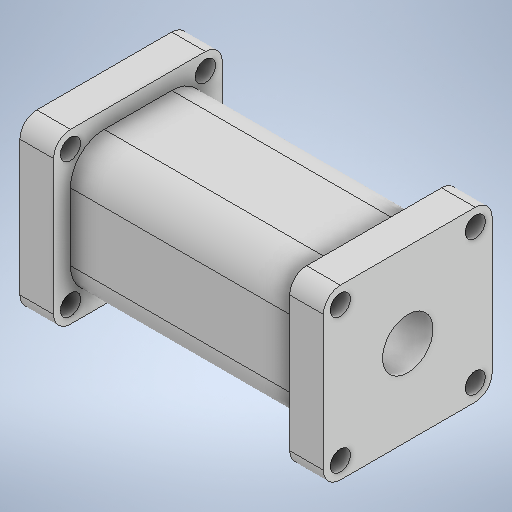
# Autodesk Inventor part: Contenedor
Saved by Autodesk Inventor 2025.1 (Build 291241000, 241)
## iProperties
Created: 2025-02-26
Part Number: Contenedor
Material: Generic
Document SubType Name: Modeling
Designer: yovan
Density: 1 g/cm^3
Appearance: Default
Author: yovan
Autodesk Inventor part; units mm, degrees
ref_plane "YZ Plane" through (0, 0, 0) normal (1, 0, 0) x (0, 1, 0)
ref_plane "XZ Plane" through (0, 0, 0) normal (0, 1, 0) x (-1, 0, 0)
ref_plane "XY Plane" through (0, 0, 0) normal (0, 0, 1) x (1, 0, 0)
sketch "Sketch1" plane through (0, 0, 0) normal (1, 0, 0) x (0, 1, 0)
  line L0 (0, 0) -> (50, 0)
  line L1 (50, 0) -> (50, 50)
  line L2 (50, 50) -> (0, 50)
  line L3 (0, 50) -> (0, 0)
  circle A0 centre (25, 25) radius 7.5
  dimension "d0" = 50
  dimension "d1" = 50
  dimension "d2" = 15
  constraints: 8 end point, 2 parallel, 1 centre point, 1 horizontal, 1 perpendicular
  measures "d0" distance of L2.end L1.end
  measures "d1" distance of L1.end L0.end
  measures "d2" diameter of A0
extrude "Extrusion1" add sketch "Sketch1" along normal blind 80
extrude "Extrusion2" add sketch "Sketch1" against normal blind 10 contours L3 L2 L1 L0 | A0
sketch "Sketch2" plane through (80, 0, 50) normal (0, 0, 1) x (1, 0, 0)
  line L0 (0, 50) -> (-90, 50) projected
  line L1 (-90, 0) -> (0, 0) projected
  line L2 (-80, 50) -> (-10, 50)
  line L3 (-10, 50) -> (-10, 0)
  line L4 (-10, 0) -> (-80, 0)
  line L5 (-80, 0) -> (-80, 50)
  line L6 (-80, 50) -> (-10, 50)
  line L7 (-10, 50) -> (-10, 45)
  line L8 (-10, 45) -> (-80, 45)
  line L9 (-80, 45) -> (-80, 50)
  line L10 (-10, 0) -> (-80, 0)
  line L11 (-80, 0) -> (-80, 5)
  line L12 (-80, 5) -> (-10, 5)
  line L13 (-10, 5) -> (-10, 0)
  point P0 (-10, 45)
  dimension "d7" = 70
  dimension "d8" = 70
  dimension "d9" = 5
  dimension "d10" = 70
  dimension "d11" = 5
  constraints: 24 end point, 6 parallel, 3 horizontal, 3 perpendicular, 2 point on line
  measures "d7" distance of L3.end L4.end
  measures "d8" distance of L7.end L8.end
  measures "d9" distance of L6.end L7.end
  measures "d10" distance of L11.end L12.end
  measures "d11" distance of L10.end L11.end
extrude "Extrusion3" cut sketch "Sketch2" against normal blind 50 contours L3 L8 L5 L0 | L3 L1 L5 L12
extrude "Extrusion4" cut sketch "Sketch2" against normal blind 5 contours L3 L12 L5 L8
sketch "Sketch3" plane through (80, 0, 0) normal (0, 0, -1) x (-1, 0, 0)
  line L0 (80, 45) -> (10, 45) projected
  line L1 (80, 5) -> (80, 0) projected
  line L2 (10, 45) -> (80, 45)
  line L3 (80, 45) -> (80, 5)
  line L4 (80, 5) -> (10, 5)
  line L5 (10, 5) -> (10, 45)
  constraints: 8 end point, 2 parallel, 1 horizontal, 1 perpendicular
extrude "Extrusion5" cut sketch "Sketch3" against normal blind 5
fillet "Fillet2" radius 5 8 edges at (-5, 50, 50) (75, 50, 50) (75, 50, 0) (-5, 50, 0) (-5, 0, 0) (75, 0, 0) (-5, 0, 50) (75, 0, 50)
fillet "Fillet3" radius 10 4 edges at (35, 45, 45) (35, 5, 45) (35, 45, 5) (35, 5, 5)
sketch "Sketch5" plane through (80, 0, 0) normal (1, 0, 0) x (0, 0, -1)
  arc A0 (-45, 50) -> (-50, 45) centre (-45, 45) ccw projected
  circle A1 centre (-45, 45) radius 3
  arc A2 (0, 45) -> (-5, 50) centre (-5, 45) ccw projected
  circle A3 centre (-5, 45) radius 3
  arc A4 (-5, 0) -> (0, 5) centre (-5, 5) ccw projected
  circle A5 centre (-5, 5) radius 3
  arc A6 (-50, 5) -> (-45, 0) centre (-45, 5) ccw projected
  circle A7 centre (-45, 5) radius 3
  point P0 (0, 0)
  dimension "d25" = 6
  dimension "d26" = 6
  dimension "d27" = 6
  dimension "d28" = 6
  constraints: 4 centre point, 4 coincident
  measures "d25" diameter of A1
  measures "d26" diameter of A3
  measures "d27" diameter of A5
  measures "d28" diameter of A7
extrude "Extrusion6" cut sketch "Sketch5" against normal blind 90
body "Solid1"
